Autodesk Fusion 360 part; units mm, degrees
(part 14 of 14)
  line L6377 (16.002, 17.4752) -> (14.986, 17.4752)
  line L6378 (20.9042, 11.049) -> (20.9042, 12.065)
  line L6379 (83.862, 28.24) -> (82.762, 28.24)
  line L6380 (24.4168, 12.198) -> (24.4168, 11.182)
  line L6381 (21.5138, 11.049) -> (20.9042, 11.049)
  line L6382 (20.9042, 11.432) -> (21.5138, 11.432)
  line L6383 (21.5138, 11.432) -> (21.5138, 11.682)
  line L6384 (82.762, 27.64) -> (83.862, 27.64)
  line L6385 (16.002, 18.0848) -> (16.002, 17.4752)
  line L6386 (20.909, 12.107) -> (20.909, 11.007)
  line L6387 (16.044, 18.08) -> (14.944, 18.08)
  line L6388 (20.9042, 12.065) -> (21.5138, 12.065)
  line L6389 (21.509, 12.107) -> (20.909, 12.107)
  line L6390 (20.9042, 11.682) -> (20.9042, 11.432)
  line L6391 (83.82, 27.6352) -> (82.804, 27.6352)
  line L6392 (82.804, 28.2448) -> (83.82, 28.2448)
  line L6393 (83.862, 27.64) -> (83.862, 28.24)
  line L6394 (21.5138, 12.065) -> (21.5138, 11.049)
  line L6395 (83.187, 28.2448) -> (83.187, 27.6352)
  line L6396 (83.187, 27.6352) -> (83.437, 27.6352)
  line L6397 (83.82, 28.2448) -> (83.82, 27.6352)
  line L6398 (16.002, 18.0848) -> (16.002, 17.4752)
  line L6399 (83.437, 28.2448) -> (83.187, 28.2448)
  line L6400 (14.986, 18.0848) -> (16.002, 18.0848)
  line L6401 (83.437, 27.6352) -> (83.437, 28.2448)
  line L6402 (14.986, 17.4752) -> (14.986, 18.0848)
  line L6403 (16.002, 17.4752) -> (14.986, 17.4752)
  line L6404 (24.412, 11.14) -> (24.412, 12.24)
  line L6405 (21.5138, 11.682) -> (20.9042, 11.682)
  line L6406 (14.986, 18.0848) -> (16.002, 18.0848)
  line L6407 (21.5138, 11.049) -> (20.9042, 11.049)
  line L6408 (82.804, 28.2448) -> (83.82, 28.2448)
  line L6409 (21.5138, 12.065) -> (21.5138, 11.049)
  line L6410 (14.944, 18.08) -> (14.944, 17.48)
  line L6411 (14.986, 17.4752) -> (14.986, 18.0848)
  line L6412 (15.113, 24.0792) -> (15.113, 24.6888)
  line L6413 (15.369, 17.4752) -> (15.619, 17.4752)
  line L6414 (20.9042, 11.049) -> (20.9042, 12.065)
  line L6415 (23.8072, 12.198) -> (24.4168, 12.198)
  line L6416 (15.113, 24.0792) -> (15.113, 24.6888)
  line L6417 (15.113, 24.6888) -> (16.129, 24.6888)
  line L6418 (24.4168, 11.815) -> (23.8072, 11.815)
  line L6419 (15.73, 19.8688) -> (15.73, 19.2592)
  line L6420 (18.3642, 25.906) -> (18.3642, 25.656)
  line L6421 (15.73, 19.2592) -> (14.714, 19.2592)
  line L6422 (24.4168, 11.182) -> (23.8072, 11.182)
  line L6423 (23.8072, 11.182) -> (23.8072, 12.198)
  line L6424 (18.9738, 26.289) -> (18.9738, 25.273)
  line L6425 (18.3642, 26.289) -> (18.9738, 26.289)
  line L6426 (15.772, 19.864) -> (14.672, 19.864)
  line L6427 (14.672, 19.264) -> (15.772, 19.264)
  line L6428 (15.113, 24.6888) -> (16.129, 24.6888)
  line L6429 (16.129, 24.0792) -> (15.113, 24.0792)
  line L6430 (24.4168, 12.198) -> (24.4168, 11.182)
  line L6431 (18.9738, 25.273) -> (18.3642, 25.273)
  line L6432 (18.9738, 25.656) -> (18.9738, 25.906)
  line L6433 (18.969, 25.231) -> (18.969, 26.331)
  line L6434 (15.746, 24.0792) -> (15.746, 24.6888)
  line L6435 (14.714, 19.8688) -> (15.73, 19.8688)
  line L6436 (15.347, 19.8688) -> (15.097, 19.8688)
  line L6437 (23.8072, 12.198) -> (24.4168, 12.198)
  line L6438 (15.097, 19.2592) -> (15.347, 19.2592)
  line L6439 (15.097, 19.8688) -> (15.097, 19.2592)
  line L6440 (16.171, 24.084) -> (16.171, 24.684)
  line L6441 (15.347, 19.2592) -> (15.347, 19.8688)
  line L6442 (14.714, 19.2592) -> (14.714, 19.8688)
  line L6443 (15.73, 19.2592) -> (14.714, 19.2592)
  arc A4220 (83.843, 27.1767) -> (83.843, 27.1132) centre (83.843, 27.145) ccw
  line L6444 (77.258, 51.643) -> (77.258, 52.243)
  line L6445 (83.843, 26.195) -> (83.843, 27.145)
  line L6446 (83.8708, 26.3398) -> (83.8708, 27.0002)
  line L6447 (83.543, 26.195) -> (83.843, 26.195)
  arc A4221 (83.843, 27.1132) -> (83.843, 27.1767) centre (83.843, 27.145) ccw
  line L6448 (20.024, 6.05) -> (21.124, 6.05)
  line L6449 (21.082, 6.0452) -> (20.066, 6.0452)
  line L6450 (20.699, 6.6548) -> (20.449, 6.6548)
  line L6451 (21.082, 5.5118) -> (21.082, 4.9022)
  line L6452 (20.066, 3.7592) -> (20.066, 4.3688)
  line L6453 (21.082, 6.6548) -> (21.082, 6.0452)
  line L6454 (21.124, 6.05) -> (21.124, 6.65)
  line L6455 (20.699, 4.9022) -> (20.699, 5.5118)
  line L6456 (20.066, 4.3688) -> (21.082, 4.3688)
  line L6457 (20.066, 6.6548) -> (21.082, 6.6548)
  line L6458 (34.802, 34.2258) -> (35.818, 34.2258)
  line L6459 (21.082, 3.7592) -> (20.066, 3.7592)
  line L6460 (20.699, 6.0452) -> (20.699, 6.6548)
  line L6461 (20.449, 6.6548) -> (20.449, 6.0452)
  line L6462 (20.066, 5.5118) -> (21.082, 5.5118)
  line L6463 (20.066, 6.0452) -> (20.066, 6.6548)
  line L6464 (20.066, 6.0452) -> (20.066, 6.6548)
  line L6465 (21.082, 4.3688) -> (21.082, 3.7592)
  line L6466 (20.449, 5.5118) -> (20.449, 4.9022)
  line L6467 (20.066, 5.5118) -> (21.082, 5.5118)
  line L6468 (35.435, 33.6162) -> (35.435, 34.2258)
  line L6469 (20.066, 4.3688) -> (21.082, 4.3688)
  line L6470 (20.449, 6.0452) -> (20.699, 6.0452)
  line L6471 (20.066, 6.6548) -> (21.082, 6.6548)
  line L6472 (42.245, 45) -> (42.245, 43.9)
  line L6473 (42.2402, 43.942) -> (42.2402, 44.958)
  line L6474 (21.082, 4.9022) -> (20.066, 4.9022)
  line L6475 (10.465, 8.388) -> (13.665, 8.388)
  line L6476 (13.7668, 8.9408) -> (10.3632, 8.9408)
  line L6477 (21.124, 7.193) -> (21.124, 7.793)
  line L6478 (20.024, 7.793) -> (20.024, 7.193)
  line L6479 (42.845, 43.9) -> (42.845, 45)
  line L6480 (42.8498, 43.942) -> (42.2402, 43.942)
  line L6481 (42.2402, 44.958) -> (42.8498, 44.958)
  line L6482 (21.082, 7.7978) -> (21.082, 7.1882)
  line L6483 (10.3632, 8.9408) -> (10.3632, 2.2352)
  line L6484 (42.8498, 44.958) -> (42.8498, 43.942)
  line L6485 (20.066, 7.7978) -> (21.082, 7.7978)
  line L6486 (10.3632, 8.9408) -> (10.3632, 2.2352)
  line L6487 (20.449, 7.1882) -> (20.699, 7.1882)
  line L6488 (20.066, 7.7978) -> (21.082, 7.7978)
  line L6489 (13.7668, 2.2352) -> (13.7668, 8.9408)
  line L6490 (21.082, 7.7978) -> (21.082, 7.1882)
  line L6491 (42.245, 43.9) -> (42.845, 43.9)
  line L6492 (20.066, 7.1882) -> (20.066, 7.7978)
  line L6493 (42.2402, 43.942) -> (42.2402, 44.958)
  line L6494 (42.8498, 44.958) -> (42.8498, 43.942)
  line L6495 (20.699, 7.7978) -> (20.449, 7.7978)
  line L6496 (42.2402, 44.325) -> (42.8498, 44.325)
  line L6497 (42.2402, 44.958) -> (42.8498, 44.958)
  line L6498 (10.3632, 2.2352) -> (13.7668, 2.2352)
  line L6499 (20.066, 7.1882) -> (20.066, 7.7978)
  line L6500 (42.8498, 44.575) -> (42.2402, 44.575)
  line L6501 (20.699, 7.1882) -> (20.699, 7.7978)
  line L6502 (42.2402, 44.575) -> (42.2402, 44.325)
  line L6503 (60.071, 8.4582) -> (59.055, 8.4582)
  line L6504 (61.299, 8.463) -> (62.399, 8.463)
  line L6505 (62.399, 8.463) -> (62.399, 9.063)
  line L6506 (10.465, 8.388) -> (13.665, 8.388)
  line L6507 (21.082, 7.1882) -> (20.066, 7.1882)
  line L6508 (42.8498, 44.325) -> (42.8498, 44.575)
  line L6509 (10.465, 2.788) -> (13.665, 2.788)
  line L6510 (10.3632, 2.2352) -> (13.7668, 2.2352)
  line L6511 (20.449, 3.7592) -> (20.699, 3.7592)
  line L6512 (42.845, 45) -> (42.245, 45)
  line L6513 (20.024, 7.193) -> (21.124, 7.193)
  line L6514 (59.688, 8.4582) -> (59.688, 9.0678)
  line L6515 (60.071, 9.0678) -> (60.071, 8.4582)
  line L6516 (62.357, 9.0678) -> (62.357, 8.4582)
  line L6517 (61.974, 9.0678) -> (61.724, 9.0678)
  line L6518 (61.341, 8.4582) -> (61.341, 9.0678)
  line L6519 (20.449, 7.7978) -> (20.449, 7.1882)
  line L6520 (42.8498, 43.942) -> (42.2402, 43.942)
  line L6521 (21.082, 7.1882) -> (20.066, 7.1882)
  line L6522 (21.124, 7.793) -> (20.024, 7.793)
  line L6523 (59.055, 9.0678) -> (60.071, 9.0678)
  line L6524 (13.7668, 8.9408) -> (10.3632, 8.9408)
  line L6525 (10.465, 8.388) -> (13.665, 8.388)
  line L6526 (13.7668, 2.2352) -> (13.7668, 8.9408)
  line L6527 (52.151, 56.473) -> (52.751, 56.473)
  line L6528 (59.013, 9.063) -> (59.013, 8.463)
  line L6529 (59.055, 8.4582) -> (59.055, 9.0678)
  line L6530 (62.399, 9.063) -> (61.299, 9.063)
  line L6531 (59.438, 8.4582) -> (59.688, 8.4582)
  line L6532 (52.151, 57.573) -> (52.151, 56.473)
  line L6533 (59.055, 8.4582) -> (59.055, 9.0678)
  line L6534 (52.1462, 57.531) -> (52.7558, 57.531)
  line L6535 (52.7558, 57.531) -> (52.7558, 56.515)
  line L6536 (59.013, 8.463) -> (60.113, 8.463)
  line L6537 (59.688, 9.0678) -> (59.438, 9.0678)
  line L6538 (10.465, 2.788) -> (13.665, 2.788)
  line L6539 (52.7558, 57.531) -> (52.7558, 56.515)
  line L6540 (62.357, 8.4582) -> (61.341, 8.4582)
  line L6541 (61.974, 8.4582) -> (61.974, 9.0678)
  line L6542 (61.299, 9.063) -> (61.299, 8.463)
  line L6543 (52.1462, 56.515) -> (52.1462, 57.531)
  line L6544 (52.1462, 57.531) -> (52.7558, 57.531)
  line L6545 (52.7558, 57.148) -> (52.1462, 57.148)
  line L6546 (59.055, 9.0678) -> (60.071, 9.0678)
  line L6547 (52.7558, 56.515) -> (52.1462, 56.515)
  line L6548 (52.1462, 57.148) -> (52.1462, 56.898)
  line L6549 (52.7558, 56.898) -> (52.7558, 57.148)
  line L6550 (10.465, 2.788) -> (13.665, 2.788)
  line L6551 (59.438, 9.0678) -> (59.438, 8.4582)
  line L6552 (52.1462, 56.898) -> (52.7558, 56.898)
  line L6553 (61.724, 9.0678) -> (61.724, 8.4582)
  line L6554 (62.357, 8.4582) -> (61.341, 8.4582)
  line L6555 (14.986, 16.3322) -> (14.986, 16.9418)
  line L6556 (60.071, 9.0678) -> (60.071, 8.4582)
  line L6557 (60.113, 8.463) -> (60.113, 9.063)
  line L6558 (61.341, 9.0678) -> (62.357, 9.0678)
  line L6559 (52.751, 57.573) -> (52.151, 57.573)
  line L6560 (52.751, 56.473) -> (52.751, 57.573)
  line L6561 (60.113, 9.063) -> (59.013, 9.063)
  line L6562 (62.357, 9.0678) -> (62.357, 8.4582)
  line L6563 (52.7558, 56.515) -> (52.1462, 56.515)
  line L6564 (52.1462, 56.515) -> (52.1462, 57.531)
  line L6565 (60.071, 8.4582) -> (59.055, 8.4582)
  line L6566 (61.341, 9.0678) -> (62.357, 9.0678)
  line L6567 (61.724, 8.4582) -> (61.974, 8.4582)
  line L6568 (61.341, 8.4582) -> (61.341, 9.0678)
  line L6569 (55.2958, 56.515) -> (54.6862, 56.515)
  line L6570 (57.231, 57.573) -> (57.231, 56.473)
  line L6571 (57.8358, 57.531) -> (57.8358, 56.515)
  line L6572 (14.986, 16.3322) -> (14.986, 16.9418)
  line L6573 (57.8358, 57.531) -> (57.8358, 56.515)
  line L6574 (14.944, 16.337) -> (16.044, 16.337)
  line L6575 (16.002, 16.3322) -> (14.986, 16.3322)
  line L6576 (14.986, 16.9418) -> (16.002, 16.9418)
  line L6577 (57.831, 56.473) -> (57.831, 57.573)
  line L6578 (55.291, 56.473) -> (55.291, 57.573)
  line L6579 (57.2262, 56.515) -> (57.2262, 57.531)
  line L6580 (55.291, 57.573) -> (54.691, 57.573)
  line L6581 (54.6862, 56.515) -> (54.6862, 57.531)
  line L6582 (16.044, 16.937) -> (14.944, 16.937)
  line L6583 (16.044, 16.337) -> (16.044, 16.937)
  line L6584 (16.002, 16.9418) -> (16.002, 16.3322)
  line L6585 (54.6862, 57.148) -> (54.6862, 56.898)
  line L6586 (57.2262, 56.898) -> (57.8358, 56.898)
  line L6587 (54.6862, 57.531) -> (55.2958, 57.531)
  line L6588 (16.002, 16.3322) -> (14.986, 16.3322)
  line L6589 (55.2958, 57.531) -> (55.2958, 56.515)
  line L6590 (57.2262, 57.531) -> (57.8358, 57.531)
  line L6591 (15.369, 16.9418) -> (15.369, 16.3322)
  line L6592 (15.619, 16.9418) -> (15.369, 16.9418)
  line L6593 (57.2262, 57.148) -> (57.2262, 56.898)
  line L6594 (15.369, 16.3322) -> (15.619, 16.3322)
  line L6595 (55.2958, 57.531) -> (55.2958, 56.515)
  line L6596 (14.986, 16.9418) -> (16.002, 16.9418)
  line L6597 (54.691, 56.473) -> (55.291, 56.473)
  line L6598 (57.2262, 57.531) -> (57.8358, 57.531)
  line L6599 (57.2262, 56.515) -> (57.2262, 57.531)
  line L6600 (55.2958, 56.515) -> (54.6862, 56.515)
  line L6601 (54.6862, 56.515) -> (54.6862, 57.531)
  line L6602 (57.8358, 56.515) -> (57.2262, 56.515)
  line L6603 (57.8358, 57.148) -> (57.2262, 57.148)
  line L6604 (16.002, 16.9418) -> (16.002, 16.3322)
  line L6605 (54.691, 57.573) -> (54.691, 56.473)
  line L6606 (15.619, 16.3322) -> (15.619, 16.9418)
  line L6607 (54.6862, 56.898) -> (55.2958, 56.898)
  line L6608 (54.6862, 57.531) -> (55.2958, 57.531)
  line L6609 (57.831, 57.573) -> (57.231, 57.573)
  line L6610 (57.8358, 56.515) -> (57.2262, 56.515)
  line L6611 (57.8358, 56.898) -> (57.8358, 57.148)
  line L6612 (57.231, 56.473) -> (57.831, 56.473)
  line L6613 (21.082, 4.9022) -> (20.066, 4.9022)
  line L6614 (20.699, 4.3688) -> (20.449, 4.3688)
  line L6615 (20.699, 5.5118) -> (20.449, 5.5118)
  line L6616 (20.699, 3.7592) -> (20.699, 4.3688)
  line L6617 (20.024, 3.764) -> (21.124, 3.764)
  line L6618 (21.124, 3.764) -> (21.124, 4.364)
  line L6619 (20.066, 3.7592) -> (20.066, 4.3688)
  line L6620 (21.082, 3.7592) -> (20.066, 3.7592)
  line L6621 (21.124, 4.364) -> (20.024, 4.364)
  line L6622 (21.082, 4.3688) -> (21.082, 3.7592)
  line L6623 (20.449, 4.3688) -> (20.449, 3.7592)
  line L6624 (20.024, 4.364) -> (20.024, 3.764)
  line L6625 (20.024, 4.907) -> (21.124, 4.907)
  line L6626 (83.8708, 27.0002) -> (83.5152, 27.0002)
sketch "micro outline" plane through (0, 0, 0) normal (0, 0, 1) x (1, 0, 0)
  line L0 (0, 63.5) -> (0, 0)
  line L1 (101.6, 63.5) -> (0, 63.5)
  line L2 (101.6, 0) -> (101.6, 63.5)
  line L3 (0, 0) -> (101.6, 0)
  line L4 (-3.81, 11.7094) -> (10.16, 11.7094)
  line L5 (-3.81, 20.5994) -> (-3.81, 11.7094)
  line L6 (10.16, 20.5994) -> (-3.81, 20.5994)
  line L7 (-5.2752, 25.77) -> (4.9948, 25.77)
  line L8 (-5.2752, 37.77) -> (-5.2752, 25.77)
  line L9 (4.7648, 37.77) -> (-5.2752, 37.77)
  arc A0 (6.35, 54.61) -> (6.35, 59.69) centre (6.35, 57.15) ccw
  arc A1 (6.35, 59.69) -> (6.35, 54.61) centre (6.35, 57.15) ccw
  arc A2 (6.35, 55.88) -> (6.35, 58.42) centre (6.35, 57.15) ccw
  arc A3 (6.35, 58.42) -> (6.35, 55.88) centre (6.35, 57.15) ccw
  arc A4 (6.35, 5.08) -> (6.35, 7.62) centre (6.35, 6.35) ccw
  arc A5 (6.35, 7.62) -> (6.35, 5.08) centre (6.35, 6.35) ccw
  arc A6 (6.35, 8.89) -> (6.35, 3.81) centre (6.35, 6.35) ccw
  arc A7 (6.35, 3.81) -> (6.35, 8.89) centre (6.35, 6.35) ccw
  arc A8 (88.9, 5.08) -> (88.9, 7.62) centre (88.9, 6.35) ccw
  arc A9 (88.9, 7.62) -> (88.9, 5.08) centre (88.9, 6.35) ccw
  arc A10 (88.9, 8.89) -> (88.9, 3.81) centre (88.9, 6.35) ccw
  arc A11 (88.9, 3.81) -> (88.9, 8.89) centre (88.9, 6.35) ccw
  line L10 (110.617, 12.446) -> (105.918, 12.446)
  line L11 (111.125, 5.842) -> (111.125, 11.938)
  line L12 (105.156, 11.684) -> (103.632, 11.684)
  line L13 (103.251, 13.843) -> (96.774, 13.843)
  line L14 (103.251, 12.065) -> (103.251, 13.843)
  line L15 (101.6, 4.064) -> (103.251, 4.064)
  line L16 (103.251, 4.064) -> (103.251, 5.715)
  line L17 (103.632, 6.096) -> (105.156, 6.096)
  line L18 (105.918, 5.334) -> (110.617, 5.334)
  line L19 (105.918, 20.574) -> (110.617, 20.574)
  line L20 (103.632, 21.336) -> (105.156, 21.336)
  line L21 (101.6, 19.304) -> (103.251, 19.304)
  line L22 (103.251, 19.304) -> (103.251, 20.955)
  line L23 (111.125, 21.082) -> (111.125, 27.178)
  line L24 (110.617, 27.686) -> (105.918, 27.686)
  line L25 (105.156, 26.924) -> (103.632, 26.924)
  line L26 (103.251, 29.083) -> (101.6, 29.083)
  line L27 (103.251, 27.305) -> (103.251, 29.083)
  line L28 (103.251, 43.688) -> (96.774, 43.688)
  line L29 (103.251, 41.91) -> (103.251, 43.688)
  line L30 (103.251, 33.909) -> (103.251, 35.56)
  line L31 (96.774, 33.909) -> (103.251, 33.909)
  line L32 (105.918, 35.179) -> (110.617, 35.179)
  line L33 (103.632, 35.941) -> (105.156, 35.941)
  line L34 (105.156, 41.529) -> (103.632, 41.529)
  line L35 (110.617, 42.291) -> (105.918, 42.291)
  line L36 (111.125, 35.687) -> (111.125, 41.783)
  line L37 (111.125, 50.927) -> (111.125, 57.023)
  line L38 (105.918, 50.419) -> (110.617, 50.419)
  line L39 (110.617, 57.531) -> (105.918, 57.531)
  line L40 (105.156, 56.769) -> (103.632, 56.769)
  line L41 (103.632, 51.181) -> (105.156, 51.181)
  line L42 (96.774, 49.149) -> (103.251, 49.149)
  line L43 (103.251, 58.928) -> (101.6, 58.928)
  line L44 (103.251, 58.928) -> (96.774, 58.928)
  line L45 (103.251, 57.15) -> (103.251, 58.928)
  line L46 (103.251, 49.149) -> (103.251, 50.8)
  arc A12 (88.9, 55.88) -> (88.9, 58.42) centre (88.9, 57.15) ccw
  arc A13 (88.9, 58.42) -> (88.9, 55.88) centre (88.9, 57.15) ccw
  arc A14 (88.9, 59.69) -> (88.9, 54.61) centre (88.9, 57.15) ccw
  arc A15 (88.9, 54.61) -> (88.9, 59.69) centre (88.9, 57.15) ccw
  arc A16 (89.5414, 57.15) -> (88.2587, 57.15) centre (88.9, 57.15) ccw
  arc A17 (88.2587, 57.15) -> (89.5414, 57.15) centre (88.9, 57.15) ccw
  arc A18 (88.2587, 6.35) -> (89.5414, 6.35) centre (88.9, 6.35) ccw
  arc A19 (89.5414, 6.35) -> (88.2587, 6.35) centre (88.9, 6.35) ccw
  arc A20 (6.9913, 6.35) -> (5.7086, 6.35) centre (6.35, 6.35) ccw
  arc A21 (5.7086, 6.35) -> (6.9913, 6.35) centre (6.35, 6.35) ccw
  arc A22 (6.9913, 57.15) -> (5.7086, 57.15) centre (6.35, 57.15) ccw
  arc A23 (5.7086, 57.15) -> (6.9913, 57.15) centre (6.35, 57.15) ccw
  line L47 (103.251, 63.5) -> (155.251, 63.5) construction
  line L48 (155.251, 63.5) -> (155.251, 0) construction
  line L49 (155.251, 0) -> (103.251, 0) construction
  line L50 (103.251, 0) -> (103.251, 63.5) construction
  line L51 (103.251, 49.149) -> (103.251, 58.928)
  line L52 (105.918, 50.419) -> (105.918, 57.531)
  line L53 (155.251, 57.531) -> (161.251, 57.531)
  line L54 (161.251, 57.531) -> (161.251, 50.419)
  line L55 (161.251, 50.419) -> (155.251, 50.419)
  line L56 (155.251, 50.419) -> (155.251, 57.531)
  line L57 (155.251, 42.291) -> (161.251, 42.291)
  line L58 (161.251, 42.291) -> (161.251, 35.179)
  line L59 (161.251, 35.179) -> (155.251, 35.179)
  line L60 (155.251, 35.179) -> (155.251, 42.291)
  line L61 (161.251, 20.574) -> (155.251, 20.574)
  line L62 (155.251, 20.574) -> (155.251, 27.686)
  line L63 (155.251, 27.686) -> (161.251, 27.686)
  line L64 (161.251, 27.686) -> (161.251, 20.574)
  line L65 (161.251, 5.334) -> (155.251, 5.334)
  line L66 (155.251, 5.334) -> (155.251, 12.446)
  line L67 (155.251, 12.446) -> (161.251, 12.446)
  line L68 (161.251, 12.446) -> (161.251, 5.334)
  line L69 (110.617, 42.291) -> (105.918, 42.291)
  line L70 (110.617, 27.686) -> (105.918, 27.686)
  line L71 (110.617, 12.446) -> (105.918, 12.446)
  line L72 (-3.9, 68.9) -> (157.851, 68.9)
  line L73 (157.851, 68.9) -> (157.851, -5.4)
  line L74 (157.851, -5.4) -> (-3.9, -5.4)
  line L75 (-3.9, -5.4) -> (-3.9, 68.9)
  point P0 (71.673, 24.124)
  point P1 (111.125, 11.938)
  dimension "d5" = 52
  dimension "d6" = 5.207
  dimension "d7" = 7.112
  dimension "d8" = 6
  dimension "d9" = 7.112
  dimension "d10" = 6
  dimension "d11" = 7.112
  dimension "d12" = 6
  dimension "d13" = 7.112
  dimension "d14" = 6
  dimension "d15" = 7.112
  dimension "d16" = 5.4
  dimension "d17" = 5.4
  dimension "d23" = 3.9
  dimension "d24" = 2.6
  constraint horizontal L47
  constraint vertical L48
  constraint horizontal L49
  constraint vertical L50
  constraint collinear L50 L51
  constraint collinear L1 L47
  constraint collinear L3 L49
  constraint horizontal L53
  constraint vertical L54
  constraint horizontal L55
  constraint vertical L56
  constraint horizontal L57
  constraint vertical L58
  constraint horizontal L59
  constraint vertical L60
  constraint horizontal L63
  constraint vertical L64
  constraint horizontal L61
  constraint vertical L62
  constraint horizontal L67
  constraint vertical L68
  constraint horizontal L65
  constraint vertical L66
  constraint collinear L39 L53
  constraint collinear L57 L69
  constraint collinear L63 L70
  constraint collinear L67 L71
  constraint horizontal L72
  constraint vertical L73
  constraint horizontal L74
  constraint vertical L75
  measures "d5" distance of L47.start L47.end
  measures "d6" distance of L37 L52
  measures "d7" distance of L38 L39
  measures "d8" distance of L53.start L53.end
  measures "d9" distance of L53.start L55.end
  measures "d10" distance of L57.end L57.start
  measures "d11" distance of L57.start L59.end
  measures "d12" distance of L62.end L63.end
  measures "d13" distance of L62.end L61.end
  measures "d14" distance of L67.end L66.end
  measures "d15" distance of L66.end L65.end
  measures "d16" distance of L1 L72
  measures "d17" distance of L3 L74
  measures "d23" distance of L0 L75
  measures "d24" distance of L48 L73
extrude "Extrude1" add sketch "micro outline" sketch "micro (1)" along normal blind 24 contours L0 L1 L2 L3 | L0 L1 L2 L3 L4 L5 L6 L7 L9 L42 L43 L44 L45 L46 L51 L53 L55 L56 L57 L59 L60 L61 L62 L63 L65 L66 L67 L72 L73 L74 L75 | L0 L7 L9 L75 | L2 L42 L43 L44 L45 L46 L51 | L0 L4 L5 L6 | L53 L55 L56 L73 | L65 L66 L67 L73 | L57 L59 L60 L73 | L61 L62 L63 L73 | A0 A1 | A2 A3 | A4 A5 | A6 A7 | A8 A9 | A10 A11 | A12 A13 | A14 A15 | A20 A21 | A22 A23 of sketch 2 contours A15 A312 | A232 A234 A235 A237 A238 A241 A245 A252 A259 A261 A264 A271 A272 A273 A278 A279 A286 A289 A290 A291 | A240 A253 A256 A280 A282 A287 A325 A327 | A251 A254 A255 A258 A262 A265 A269 A284 A292 A297 A300 A301 A303 A311 A313 A317 A319 A321 A324 A328 | A302 A316 makes body 1
sketch "antennas" plane through (157.851, 0, 0) normal (1, 0, 0) x (0, 1, 0)
  line L0 (-5.4, 0) -> (68.9, 0)
  line L1 (68.9, 0) -> (68.9, 24)
  line L2 (68.9, 24) -> (-5.4, 24)
  line L3 (-5.4, 24) -> (-5.4, 0)
  line L4 (12.446, 0) -> (5.334, 0)
  line L5 (27.686, 0) -> (20.574, 0)
  line L6 (42.291, 0) -> (35.179, 0)
  line L7 (57.531, 0) -> (50.419, 0)
  line L8 (8.89, 0) -> (8.89, 6.8) construction
  line L9 (24.13, 0) -> (24.13, 6.8) construction
  line L10 (38.735, 0) -> (38.735, 6.8) construction
  line L11 (53.975, 0) -> (53.975, 6.8) construction
  circle A0 centre (8.89, 6.8) radius 3.55
  circle A1 centre (24.13, 6.8) radius 3.55
  circle A2 centre (38.735, 6.8) radius 3.55
  circle A3 centre (53.975, 6.8) radius 3.55
  dimension "d33" = 6.8
  dimension "d34" = 6.8
  dimension "d35" = 6.8
  dimension "d36" = 6.8
  dimension "d37" = 7.1
  dimension "d38" = 7.1
  dimension "d39" = 7.1
  dimension "d40" = 7.1
  constraint midpoint L4 L8.start
  constraint perpendicular L4 L8
  constraint midpoint L5 L9.start
  constraint perpendicular L5 L9
  constraint midpoint L6 L10.start
  constraint perpendicular L6 L10
  constraint midpoint L7 L11.start
  constraint perpendicular L7 L11
  constraint coincident L8.end A0.centre
  constraint coincident L9.end A1.centre
  constraint coincident L10.end A2.centre
  constraint coincident L11.end A3.centre
  measures "d33" distance of L8.start L8.end
  measures "d34" distance of L9.start L9.end
  measures "d35" distance of L10.start L10.end
  measures "d36" distance of L11.start L11.end
  measures "d37" diameter of A0
  measures "d38" diameter of A1
  measures "d39" diameter of A2
  measures "d40" diameter of A3
ref_plane "WorkPlane1" through (76.9755, 31.75, 8) normal (0, 0, -1) x (-1, 0, 0)
split "Split1" by plane through (76.9755, 31.75, 8) normal (0, 0, -1) bodies 1 makes body 2 at (50.017, 44.1333, 0)
shell "Shell1" thickness 2 removed faces 1 at (103.934, 44.1333, 8) on bodies 2
shell "Shell2" thickness 2 removed faces 1 at (103.934, 44.1333, 8) on bodies 1
sketch "power" plane through (0, 0, 8) normal (0, 0, -1) x (1, 0, 0)
  line L0 (-3.9, 5.4) -> (-3.9, -68.9)
  line L1 (-3.9, -68.9) -> (157.851, -68.9)
  line L2 (157.851, -68.9) -> (157.851, 5.4)
  line L3 (157.851, 5.4) -> (-3.9, 5.4)
  line L4 (-3.81, -11.7094) -> (10.16, -11.7094)
  line L5 (-3.81, -20.5994) -> (-3.81, -11.7094)
  line L6 (10.16, -20.5994) -> (-3.81, -20.5994)
  line L7 (-5.2752, -25.77) -> (4.9948, -25.77)
  line L8 (-5.2752, -37.77) -> (-5.2752, -25.77)
  line L9 (4.7648, -37.77) -> (-5.2752, -37.77)
  line L10 (155.251, -20.574) -> (155.251, -27.686)
  line L11 (161.251, -27.686) -> (161.251, -20.574)
  line L12 (155.251, -27.686) -> (161.251, -27.686)
  line L13 (161.251, -20.574) -> (155.251, -20.574)
  line L14 (155.251, -5.334) -> (155.251, -12.446)
  line L15 (161.251, -12.446) -> (161.251, -5.334)
  line L16 (161.251, -5.334) -> (155.251, -5.334)
  line L17 (155.251, -12.446) -> (161.251, -12.446)
  line L18 (155.251, -35.179) -> (155.251, -42.291)
  line L19 (155.251, -42.291) -> (161.251, -42.291)
  line L20 (161.251, -35.179) -> (155.251, -35.179)
  line L21 (161.251, -42.291) -> (161.251, -35.179)
  line L22 (155.251, -50.419) -> (155.251, -57.531)
  line L23 (155.251, -57.531) -> (161.251, -57.531)
  line L24 (161.251, -50.419) -> (155.251, -50.419)
  line L25 (161.251, -57.531) -> (161.251, -50.419)
  line L26 (-3.9, -11.2094) -> (0.1, -11.2094)
  line L27 (0.1, -11.2094) -> (0.1, -21.0994)
  line L28 (0.1, -21.0994) -> (-3.9, -21.0994)
  line L29 (-3.9, -21.0994) -> (-3.9, -11.2094)
  line L30 (-3.9, -25.27) -> (0.1, -25.27)
  line L31 (0.1, -25.27) -> (0.1, -38.27)
  line L32 (0.1, -38.27) -> (-3.9, -38.27)
  line L33 (-3.9, -38.27) -> (-3.9, -25.27)
  line L34 (-1.9, 3.4) -> (155.851, 3.4)
  line L35 (155.851, 3.4) -> (155.851, -66.9)
  line L36 (155.851, -66.9) -> (-1.9, -66.9)
  line L37 (-1.9, -66.9) -> (-1.9, 3.4)
  dimension "d25" = 0.5
  dimension "d26" = 0.5
  dimension "d27" = 0.5
  dimension "d28" = 0.5
  constraint horizontal L26
  constraint vertical L27
  constraint horizontal L28
  constraint vertical L29
  constraint coincident L0 L26.start
  constraint horizontal L30
  constraint vertical L31
  constraint horizontal L32
  constraint vertical L33
  constraint coincident L0 L30.start
  measures "d25" distance of L4 L26
  measures "d26" distance of L6 L28
  measures "d27" distance of L7 L30
  measures "d28" distance of L9 L32
sketch "lip" plane through (0, 0, 8) normal (0, 0, 1) x (-1, 0, 0)
  line L0 (-155.851, -66.9) -> (-155.851, 3.4)
  line L1 (-155.851, 3.4) -> (1.9, 3.4)
  line L2 (1.9, 3.4) -> (1.9, -66.9)
  line L3 (1.9, -66.9) -> (-155.851, -66.9)
  line L4 (3.9, -68.9) -> (3.9, 5.4)
  line L5 (3.9, 5.4) -> (-157.851, 5.4)
  line L6 (-157.851, 5.4) -> (-157.851, -68.9)
  line L7 (-157.851, -68.9) -> (3.9, -68.9)
  line L8 (2.9, -67.9) -> (-156.851, -67.9)
  line L9 (-156.851, -67.9) -> (-156.851, 4.4)
  line L10 (-156.851, 4.4) -> (2.9, 4.4)
  line L11 (2.9, 4.4) -> (2.9, -67.9)
  line L12 (-0.1, -21.0994) -> (3.9, -21.0994)
  line L13 (3.9, -11.2094) -> (-0.1, -11.2094)
  line L14 (3.9, -25.27) -> (-0.1, -25.27)
  line L15 (-0.1, -38.27) -> (3.9, -38.27)
  dimension "d57" = 1
  dimension "d58" = 1
  dimension "d59" = 1
  dimension "d60" = 1
  constraint horizontal L8
  constraint vertical L9
  constraint horizontal L10
  constraint vertical L11
  measures "d57" distance of L0 L9
  measures "d58" distance of L1 L10
  measures "d59" distance of L3 L8
  measures "d60" distance of L2 L11
extrude "Extrude9" add sketch "lip" along normal blind 2 contours L0 L1 L2 L3 L8 L9 L10 L11 L13 L15 | L2 L11 L12 L14 bodies 2
combine "Combine2" operation cut target body 1 tool bodies 2 keep tools
extrude "Extrude2" cut sketch "power" against normal blind 12.7 contours L0 L4 L5 L6 L26 L28 L29 L37 | L4 L26 L27 L37 | L6 L27 L28 L37 | L4 L5 L6 L37 | L4 L6 L27 L37 bodies 1
extrude "Extrude3" cut sketch "power" against normal blind 14.7 contours L0 L7 L30 L33 L37 | L0 L7 L9 L33 L37 | L7 L30 L31 L37 | L0 L9 L32 L33 L37 | L7 L9 L31 L37 | L9 L31 L32 L37 bodies 1
extrude "Extrude5" cut sketch "antennas" along normal mid plane 8 contours A0 | A1 | A2 | A3 bodies 1 2
fillet "Fillet1" radius 1 16 edges at (76.9755, -5.4, 24) (-3.9, 31.75, 24) (76.9755, 68.9, 24) (157.851, 31.75, 24) (157.851, -5.4, 16) (157.851, 68.9, 16) (-3.9, -5.4, 16) (-3.9, 68.9, 16) (157.851, 68.9, 4) (157.851, -5.4, 4) (-3.9, 68.9, 4) (-3.9, -5.4, 4) (-3.9, 31.75, 0) (76.9755, 68.9, 0) (76.9755, -5.4, 0) (157.851, 31.75, 0) on bodies 1 2
sketch "posts" plane through (0, 0, 2) normal (0, 0, 1) x (-1, 0, 0)
  line L0 (1.9, 3.4) -> (-155.851, 3.4)
  line L1 (-155.851, 3.4) -> (-155.851, -66.9)
  line L2 (-155.851, -66.9) -> (1.9, -66.9)
  line L3 (1.9, -66.9) -> (1.9, 3.4)
  arc A0 (-88.9, -54.61) -> (-88.9, -59.69) centre (-88.9, -57.15) ccw
  arc A1 (-88.9, -59.69) -> (-88.9, -54.61) centre (-88.9, -57.15) ccw
  arc A2 (-90.4748, -57.15) -> (-87.3252, -57.15) centre (-88.9, -57.15) ccw
  arc A3 (-87.3252, -57.15) -> (-90.4748, -57.15) centre (-88.9, -57.15) ccw
  arc A4 (-88.9, -3.81) -> (-88.9, -8.89) centre (-88.9, -6.35) ccw
  arc A5 (-88.9, -8.89) -> (-88.9, -3.81) centre (-88.9, -6.35) ccw
  arc A6 (-90.4748, -6.35) -> (-87.3252, -6.35) centre (-88.9, -6.35) ccw
  arc A7 (-87.3252, -6.35) -> (-90.4748, -6.35) centre (-88.9, -6.35) ccw
  arc A8 (-6.35, -3.81) -> (-6.35, -8.89) centre (-6.35, -6.35) ccw
  arc A9 (-6.35, -8.89) -> (-6.35, -3.81) centre (-6.35, -6.35) ccw
  arc A10 (-7.9248, -6.35) -> (-4.7752, -6.35) centre (-6.35, -6.35) ccw
  arc A11 (-4.7752, -6.35) -> (-7.9248, -6.35) centre (-6.35, -6.35) ccw
  arc A12 (-6.35, -54.61) -> (-6.35, -59.69) centre (-6.35, -57.15) ccw
  arc A13 (-6.35, -59.69) -> (-6.35, -54.61) centre (-6.35, -57.15) ccw
  arc A14 (-6.35, -55.5879) -> (-6.35, -58.7121) centre (-6.35, -57.15) ccw
  arc A15 (-6.35, -58.7121) -> (-6.35, -55.5879) centre (-6.35, -57.15) ccw
extrude "Extrude6" add sketch "posts" along normal blind 4 contours A0 A1 | A4 A5 | A8 A9 | A12 A13 bodies 2
extrude "Extrude7" cut sketch "posts" against normal up to surface (2 mm away) contours A2 A3 | A6 A7 | A10 A11 | A14 A15 bodies 2
chamfer "Chamfer1" distance 1 angle 45 4 edges at (5.4315, 54.7819, 2) (5.4315, 3.9819, 2) (87.9815, 3.9819, 2) (87.9815, 54.7819, 2) on bodies 2
fillet "Fillet2" radius 2 4 edges at (7.8182, 6.9195, 0) (90.3682, 6.9195, 0) (6.9149, 55.6936, 0) (90.3682, 57.7195, 0) on bodies 2
chamfer "Chamfer2" distance 1 angle 45 10 edges at (155.851, 31.75, 2) (76.9755, 66.9, 2) (-1.9, 31.75, 2) (76.9755, -3.4, 2) (155.851, 31.75, 22) (76.9755, -3.4, 22) (-1.9, 52.585, 22) (-1.9, 10.935, 22) (-1.9, 52.585, 22) (76.9755, 66.9, 22) on bodies 1 2
sketch "top posts and vents" plane through (0, 0, 22) normal (0, 0, -1) x (1, 0, 0)
  line L0 (-0.9, 2.4) -> (-0.9, -25.27)
  line L1 (-0.9, -25.27) -> (0.1, -25.27)
  line L2 (0.1, -25.27) -> (0.1, -38.27)
  line L3 (0.1, -38.27) -> (-0.9, -38.27)
  line L4 (-0.9, -38.27) -> (-0.9, -65.9)
  line L5 (-0.9, -65.9) -> (154.851, -65.9)
  line L6 (154.851, -65.9) -> (154.851, 2.4)
  line L7 (154.851, 2.4) -> (-0.9, 2.4)
  arc A0 (6.35, -8.89) -> (6.35, -3.81) centre (6.35, -6.35) ccw
  arc A1 (6.35, -3.81) -> (6.35, -8.89) centre (6.35, -6.35) ccw
  arc A2 (88.9, -8.89) -> (88.9, -3.81) centre (88.9, -6.35) ccw
  arc A3 (88.9, -3.81) -> (88.9, -8.89) centre (88.9, -6.35) ccw
  arc A4 (88.9, -59.69) -> (88.9, -54.61) centre (88.9, -57.15) ccw
  arc A5 (88.9, -54.61) -> (88.9, -59.69) centre (88.9, -57.15) ccw
  arc A6 (6.35, -59.69) -> (6.35, -54.61) centre (6.35, -57.15) ccw
  arc A7 (6.35, -54.61) -> (6.35, -59.69) centre (6.35, -57.15) ccw
  circle A8 centre (6.35, -6.35) radius 0.95
  circle A9 centre (88.9, -6.35) radius 0.95
  circle A10 centre (6.35, -57.15) radius 0.95
  circle A11 centre (88.9, -57.15) radius 0.95
  line L8 (77.4694, -5.7) -> (57.4694, -5.7)
  arc A12 (57.4694, -5.7) -> (57.4694, -7) centre (57.4694, -6.35) ccw
  line L9 (57.4694, -7) -> (77.4694, -7)
  arc A13 (77.4694, -7) -> (77.4694, -5.7) centre (77.4694, -6.35) ccw
  line L10 (77.4694, -6.35) -> (57.4694, -6.35) construction
  line L11 (16.4694, -7) -> (36.4694, -7)
  arc A14 (36.4694, -7) -> (36.4694, -5.7) centre (36.4694, -6.35) ccw
  arc A15 (16.4694, -5.7) -> (16.4694, -7) centre (16.4694, -6.35) ccw
  line L12 (36.4694, -5.7) -> (16.4694, -5.7)
  line L13 (57.4694, -14.2857) -> (77.4694, -14.2857)
  arc A16 (77.4694, -14.2857) -> (77.4694, -12.9857) centre (77.4694, -13.6357) ccw
  arc A17 (57.4694, -12.9857) -> (57.4694, -14.2857) centre (57.4694, -13.6357) ccw
  line L14 (77.4694, -12.9857) -> (57.4694, -12.9857)
  line L15 (16.4694, -14.2857) -> (36.4694, -14.2857)
  arc A18 (36.4694, -14.2857) -> (36.4694, -12.9857) centre (36.4694, -13.6357) ccw
  arc A19 (16.4694, -12.9857) -> (16.4694, -14.2857) centre (16.4694, -13.6357) ccw
  line L16 (36.4694, -12.9857) -> (16.4694, -12.9857)
  line L17 (57.4694, -21.5714) -> (77.4694, -21.5714)
  arc A20 (77.4694, -21.5714) -> (77.4694, -20.2714) centre (77.4694, -20.9214) ccw
  arc A21 (57.4694, -20.2714) -> (57.4694, -21.5714) centre (57.4694, -20.9214) ccw
  line L18 (77.4694, -20.2714) -> (57.4694, -20.2714)
  line L19 (16.4694, -21.5714) -> (36.4694, -21.5714)
  arc A22 (36.4694, -21.5714) -> (36.4694, -20.2714) centre (36.4694, -20.9214) ccw
  arc A23 (16.4694, -20.2714) -> (16.4694, -21.5714) centre (16.4694, -20.9214) ccw
  line L20 (36.4694, -20.2714) -> (16.4694, -20.2714)
  line L21 (57.4694, -28.8571) -> (77.4694, -28.8571)
  arc A24 (77.4694, -28.8571) -> (77.4694, -27.5571) centre (77.4694, -28.2071) ccw
  arc A25 (57.4694, -27.5571) -> (57.4694, -28.8571) centre (57.4694, -28.2071) ccw
  line L22 (77.4694, -27.5571) -> (57.4694, -27.5571)
  line L23 (16.4694, -28.8571) -> (36.4694, -28.8571)
  arc A26 (36.4694, -28.8571) -> (36.4694, -27.5571) centre (36.4694, -28.2071) ccw
  arc A27 (16.4694, -27.5571) -> (16.4694, -28.8571) centre (16.4694, -28.2071) ccw
  line L24 (36.4694, -27.5571) -> (16.4694, -27.5571)
  line L25 (57.4694, -36.1429) -> (77.4694, -36.1429)
  arc A28 (77.4694, -36.1429) -> (77.4694, -34.8429) centre (77.4694, -35.4929) ccw
  arc A29 (57.4694, -34.8429) -> (57.4694, -36.1429) centre (57.4694, -35.4929) ccw
  line L26 (77.4694, -34.8429) -> (57.4694, -34.8429)
  line L27 (16.4694, -36.1429) -> (36.4694, -36.1429)
  arc A30 (36.4694, -36.1429) -> (36.4694, -34.8429) centre (36.4694, -35.4929) ccw
  arc A31 (16.4694, -34.8429) -> (16.4694, -36.1429) centre (16.4694, -35.4929) ccw
  line L28 (36.4694, -34.8429) -> (16.4694, -34.8429)
  line L29 (57.4694, -43.4286) -> (77.4694, -43.4286)
  arc A32 (77.4694, -43.4286) -> (77.4694, -42.1286) centre (77.4694, -42.7786) ccw
  arc A33 (57.4694, -42.1286) -> (57.4694, -43.4286) centre (57.4694, -42.7786) ccw
  line L30 (77.4694, -42.1286) -> (57.4694, -42.1286)
  line L31 (16.4694, -43.4286) -> (36.4694, -43.4286)
  arc A34 (36.4694, -43.4286) -> (36.4694, -42.1286) centre (36.4694, -42.7786) ccw
  arc A35 (16.4694, -42.1286) -> (16.4694, -43.4286) centre (16.4694, -42.7786) ccw
  line L32 (36.4694, -42.1286) -> (16.4694, -42.1286)
  line L33 (57.4694, -50.7143) -> (77.4694, -50.7143)
  arc A36 (77.4694, -50.7143) -> (77.4694, -49.4143) centre (77.4694, -50.0643) ccw
  arc A37 (57.4694, -49.4143) -> (57.4694, -50.7143) centre (57.4694, -50.0643) ccw
  line L34 (77.4694, -49.4143) -> (57.4694, -49.4143)
  line L35 (16.4694, -50.7143) -> (36.4694, -50.7143)
  arc A38 (36.4694, -50.7143) -> (36.4694, -49.4143) centre (36.4694, -50.0643) ccw
  arc A39 (16.4694, -49.4143) -> (16.4694, -50.7143) centre (16.4694, -50.0643) ccw
  line L36 (36.4694, -49.4143) -> (16.4694, -49.4143)
  line L37 (57.4694, -58) -> (77.4694, -58)
  arc A40 (77.4694, -58) -> (77.4694, -56.7) centre (77.4694, -57.35) ccw
  arc A41 (57.4694, -56.7) -> (57.4694, -58) centre (57.4694, -57.35) ccw
  line L38 (77.4694, -56.7) -> (57.4694, -56.7)
  line L39 (16.4694, -58) -> (36.4694, -58)
  arc A42 (36.4694, -58) -> (36.4694, -56.7) centre (36.4694, -57.35) ccw
  arc A43 (16.4694, -56.7) -> (16.4694, -58) centre (16.4694, -57.35) ccw
  line L40 (36.4694, -56.7) -> (16.4694, -56.7)
  dimension "d64" = 1.9
  dimension "d65" = 1.9
  dimension "d66" = 1.9
  dimension "d67" = 1.9
  dimension "d73" = -41
  dimension "d74" = -51
  constraint concentric A0 A8
  constraint concentric A2 A9
  constraint concentric A6 A10
  constraint concentric A5 A11
  constraint tangent L8 A12
  constraint tangent A12 L9
  constraint parallel L8 L9
  constraint tangent L9 A13
  constraint tangent L8 A13
  constraint horizontal L10
  measures "d64" diameter of A8
  measures "d65" diameter of A9
  measures "d66" diameter of A10
  measures "d67" diameter of A11
extrude "Extrude10" add sketch "top posts and vents" along normal blind 14 contours A0 A1 | A2 A3 | A4 A5 | A6 A7 bodies 1
chamfer "Chamfer3" distance 2 angle 45 4 edges at (5.4315, 8.7181, 22) (87.9815, 8.7181, 22) (87.9815, 59.5181, 22) (5.4315, 59.5181, 22) on bodies 1
extrude "Extrude11" cut sketch "top posts and vents" against normal up to surface (2 mm away) contours L8 A12 L9 A13 | L11 A14 A15 L12 | L13 A16 A17 L14 | L15 A18 A19 L16 | L17 A20 A21 L18 | L19 A22 A23 L20 | L21 A24 A25 L22 | L23 A26 A27 L24 | L25 A28 A29 L26 | L27 A30 A31 L28 | L29 A32 A33 L30 | L31 A34 A35 L32 | L33 A36 A37 L34 | L35 A38 A39 L36 | L37 A40 A41 L38 | L39 A42 A43 L40 bodies 1
equation "d16 = 3 mm + ( ( 0.8 * 3 ) * 1 mm )"
equation "d17 = 3 mm + ( 0.8 * 3 ) * 1 mm"
equation "d23 = 1.5 mm + ( ( 0.8 * 3 ) * 1 mm )"
equation "d24 = 1 mm + ( 0.8 * 2 ) * 1 mm"
equation "d29 = ( -1 * ( 1.7 + 11 ) ) * 1 mm"
equation "d31 = ( -1 * ( 1.7 + 13 ) ) * 1 mm"
named bodies: "Top", "Bottom"
